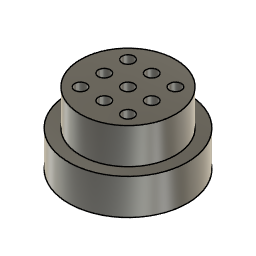
sprinkler for tube v1 (Autodesk Fusion 360 design; units mm, degrees)
Autodesk Fusion 360 part; units mm, degrees
sketch "Sketch1" plane through (0, 0, 0) normal (0, 0, 1) x (1, 0, 0)
  circle A0 centre (0, 0) radius 4
  circle A1 centre (0, 0) radius 5
  dimension "d1" = 8
  dimension "d2" = 1
  constraint coincident A0.centre A1.centre
  measures "d1" diameter of A0
extrude "Extrude1" add sketch "Sketch1" along normal blind 3
extrude "Extrude2" add sketch "Sketch1" along normal blind 6 contours A0
sketch "Sketch2" plane through (0, 0, 6) normal (0, 0, 1) x (-1, 0, 0)
  circle A0 centre (0, 0) radius 4
  circle A1 centre (-2, 2) radius 0.5
  circle A2 centre (0, 2) radius 0.5
  circle A3 centre (2, 2) radius 0.5
  circle A4 centre (-2, 0) radius 0.5
  circle A5 centre (0, 0) radius 0.5
  circle A6 centre (2, 0) radius 0.5
  circle A7 centre (-2, -2) radius 0.5
  circle A8 centre (0, -2) radius 0.5
  circle A9 centre (2, -2) radius 0.5
  point P0 (-2, 2)
  dimension "d7" = 1
  dimension "d8" = 1
  dimension "d9" = 1
  dimension "d10" = 1
  dimension "d11" = 1
  dimension "d12" = 1
  dimension "d13" = 1
  dimension "d14" = 1
  dimension "d15" = 1
  measures "d7" diameter of A1
  measures "d8" diameter of A2
  measures "d9" diameter of A3
  measures "d10" diameter of A4
  measures "d11" diameter of A5
  measures "d12" diameter of A6
  measures "d13" diameter of A7
  measures "d14" diameter of A8
  measures "d15" diameter of A9
hole "Hole1" at (2, -2, 6) at (0, -2, 6) at (-2, -2, 6) at (2, 0, 6) at (0, 0, 6) at (-2, 0, 6) at (2, 2, 6) at (0, 2, 6) at (-2, 2, 6) direction (0, 0, -1) diameter 1 depth 6 tip angle 180
